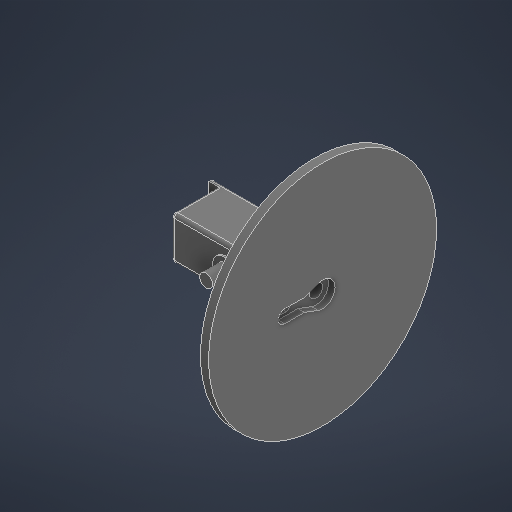
# Autodesk Inventor part: arm_MALE_full_size
Saved by Autodesk Inventor 2026.1 (Build 301233000, 233)
## iProperties
Created: 2025-10-10
Part Number: arm_MALE_full_size
Material: Generic
Document SubType Name: Modeling
Designer: Ethan
Density: 1 g/cm^3
Appearance: Gray
Author: Ethan
Autodesk Inventor part; units mm, degrees
ref_plane "YZ Plane" through (0, 0, 0) normal (1, 0, 0) x (0, 1, 0)
ref_plane "XZ Plane" through (0, 0, 0) normal (0, 1, 0) x (-1, 0, 0)
ref_plane "XY Plane" through (0, 0, 0) normal (0, 0, 1) x (1, 0, 0)
sketch "Sketch1" plane through (0, 0, 0) normal (0, 0, 1) x (1, 0, 0)
  line L0 (0, 0) -> (-40.25, 0)
  line L1 (-40.25, 0) -> (-40.25, 20.25)
  line L2 (-40.25, 20.25) -> (0, 20.25)
  line L3 (0, 20.25) -> (0, 0)
  dimension "d0" = 40.25
  dimension "d1" = 20.25
  constraints: 8 end point, 2 parallel, 1 horizontal, 1 perpendicular
  measures "d0" distance of L1.end L2.end
  measures "d1" distance of L0.end L1.end
extrude "Extrusion1" add sketch "Sketch1" along normal blind 3
sketch "Sketch2" plane through (0, 0, 3) normal (0, 0, 1) x (1, 0, 0)
  line L0 (0, 20.25) -> (-40.25, 20.25) projected
  line L1 (0, 20.25) -> (3, 20.25)
  line L2 (3, 20.25) -> (3, 14.125)
  line L3 (3, 14.125) -> (0, 14.125)
  line L4 (0, 14.125) -> (0, 20.25)
  line L5 (0, 0) -> (3, 0)
  line L6 (3, 0) -> (3, 6.125)
  line L7 (3, 6.125) -> (0, 6.125)
  line L8 (0, 6.125) -> (0, 0)
  line L9 (3, 20.25) -> (-40.25, 20.25)
  line L10 (-40.25, 20.25) -> (-40.25, 23.25)
  line L11 (-40.25, 23.25) -> (3, 23.25)
  line L12 (3, 23.25) -> (3, 20.25)
  line L13 (-40.25, 20.25) -> (-40.25, 0) projected
  line L14 (-40.25, 0) -> (-43.25, 0)
  line L15 (-43.25, 0) -> (-43.25, 23.25)
  line L16 (-43.25, 23.25) -> (-40.25, 23.25)
  line L17 (-40.25, 23.25) -> (-40.25, 0)
  line L18 (-43.25, 0) -> (3, 0)
  line L19 (3, 0) -> (3, -3)
  line L20 (3, -3) -> (-43.25, -3)
  line L21 (-43.25, -3) -> (-43.25, 0)
  point P0 (1.5, 6.125)
  dimension "d4" = 8
  dimension "d5" = 6.125
  dimension "d6" = 6.125
  dimension "d7" = 3
  dimension "d8" = 3
  dimension "d9" = 3
  dimension "d10" = 3
  dimension "d11" = 3
  constraints: 40 end point, 10 parallel, 5 horizontal, 5 perpendicular, 1 midpoint
  measures "d4" distance from line of L3 point (1.5, 6.125)
  measures "d5" distance of L1.end L2.end
  measures "d6" distance of L5.end L6.end
  measures "d7" distance between parallel lines of L4 L2
  measures "d8" distance between parallel lines of L8 L6
  measures "d9" distance between parallel lines of L0 L11
  measures "d10" distance between parallel lines of L13 L15
  measures "d11" distance between parallel lines of L18 L20
extrude "Extrusion2" add sketch "Sketch2" against normal blind 18
sketch "Sketch3" plane through (0, 0, -15) normal (0, 0, -1) x (-1, 0, 0)
  line L0 (-3, 23.25) -> (-3, 14.125) projected
  line L1 (43.25, -3) -> (43.25, 23.25) projected
  line L2 (-3, 23.25) -> (43.25, 23.25)
  line L3 (43.25, 23.25) -> (43.25, 20.25)
  line L4 (43.25, 20.25) -> (-3, 20.25)
  line L5 (-3, 20.25) -> (-3, 23.25)
  line L6 (0, 20.25) -> (40.25, 20.25) projected
  line L7 (-3, -3) -> (-3, 6.125) projected
  line L8 (-3, 0) -> (43.25, 0)
  line L9 (43.25, 0) -> (43.25, -3)
  line L10 (43.25, -3) -> (-3, -3)
  line L11 (-3, -3) -> (-3, 0)
  point P0 (0, 0)
  point P1 (-3, 20.25)
  dimension "d14" = 0
  constraints: 16 end point, 4 parallel, 2 horizontal, 2 perpendicular, 2 point on line
  measures "d14" distance between parallel lines of L6 L4
extrude "Extrusion3" add sketch "Sketch3" along normal blind 13
sketch "Sketch4" plane through (-43.25, -3, 3) normal (-1, 0, 0) x (0, 0, 1)
  line L0 (0, 0) -> (-31, 0) projected
  line L1 (-31, 26.25) -> (-28, 26.25)
  line L2 (-28, 26.25) -> (-28, 0)
  line L3 (-28, 0) -> (-31, 0)
  line L4 (-31, 0) -> (-31, 26.25)
  line L5 (0, 26.25) -> (-31, 26.25) projected
  point P0 (-3, 3)
  dimension "d17" = 3
  dimension "d18" = 0
  constraints: 8 end point, 2 parallel, 1 horizontal, 1 perpendicular, 1 point on line
  measures "d17" distance from line of L1.start L2
  measures "d18" distance between parallel lines of L1 L5
extrude "Extrusion4" add sketch "Sketch4" against normal blind 3
sketch "Sketch5" plane through (-43.25, -3, 3) normal (-1, 0, 0) x (0, 0, 1)
  line L0 (0, 26.25) -> (-31, 26.25) projected
  line L1 (0, 0) -> (-31, 0) projected
  line L2 (-31, 26.25) -> (-28, 26.25)
  line L3 (-28, 26.25) -> (-28, 0)
  line L4 (-28, 0) -> (-31, 0)
  line L5 (-31, 0) -> (-31, 26.25)
  line L6 (-28, 3) -> (-28, 23.25) projected
  point P0 (-3, 3)
  dimension "d21" = 0
  constraints: 8 end point, 2 parallel, 1 horizontal, 1 perpendicular, 1 point on line
  measures "d21" distance between parallel lines of L6 L3
extrude "Extrusion5" add sketch "Sketch5" along normal blind 5
sketch "Sketch6" plane through (0, 0, -28) normal (0, 0, -1) x (-1, 0, 0)
  circle A0 centre (44.55, 17.25) radius 2.5
  circle A1 centre (44.55, 3) radius 2.5
  line L0 (-3, 23.25) -> (48.25, 23.25) projected
  line L1 (-3, -3) -> (48.25, -3) projected
  line L2 (40.25, 0) -> (40.25, 20.25) projected
  line L3 (42.05, 17.25) -> (47.05, 17.25)
  line L4 (47.05, 17.25) -> (47.05, 3)
  line L5 (47.05, 3) -> (42.05, 3)
  line L6 (42.05, 3) -> (42.05, 17.25)
  point P0 (0, 0)
  point P1 (42.05, 3)
  point P2 (42.05, 3)
  point P3 (46.4709, 4.6)
  dimension "d26" = 5
  dimension "d27" = 5
  dimension "d24" = 6
  dimension "d25" = 6
  dimension "d28" = 4.3
  dimension "d29" = 4.3
  constraints: 8 end point, 2 parallel, 2 vertical, 1 horizontal, 1 perpendicular, 6 other
  measures "d24" distance from line of L0 point (44.55, 17.25)
  measures "d25" distance from line of L1 point (44.55, 3)
  measures "d28" distance from line of L2 point (44.55, 17.25)
  measures "d29" distance from line of L2 point (44.55, 3)
extrude "Extrusion6" cut sketch "Sketch6" against normal blind 3
sketch "Sketch7" plane through (-43.25, -3, 3) normal (-1, 0, 0) x (0, 0, 1)
  line L0 (-18, 23.25) -> (-31, 23.25) projected
  line L1 (-3, 3) -> (-18, 3) projected
  line L2 (-18, 23.25) -> (-11, 23.25)
  line L3 (-11, 23.25) -> (-11, 3)
  line L4 (-11, 3) -> (-18, 3)
  line L5 (-18, 3) -> (-18, 23.25)
  line L6 (-28, 0) -> (-28, 26.25) projected
  dimension "d38" = 17
  constraints: 8 end point, 2 parallel, 1 horizontal, 1 perpendicular, 1 point on line
  measures "d38" distance between parallel lines of L6 L3
extrude "Extrusion7" cut sketch "Sketch7" against normal blind 3
sketch "Sketch8" plane through (0, 0, 3) normal (0, 0, 1) x (1, 0, 0)
  line L0 (0, 6.125) -> (0, 14.125) projected
  line L1 (-43.25, -3) -> (3, -3) projected
  line L2 (3, 23.25) -> (-43.25, 23.25) projected
  circle A0 centre (-10, 10) radius 7
  point P0 (0, 0)
  point P1 (0, 10.125)
  point P2 (-2, 5)
  point P3 (-15, 2)
  point P4 (-18, 15)
  dimension "d69" = 14
  constraints: 1 centre point, 1 midpoint
  measures "d69" diameter of A0
extrude "Extrusion8" add sketch "Sketch8" along normal blind 1
sketch "Sketch11" plane through (-10, 10, 4) normal (0, 0, 1) x (1, 0, 0)
  circle A0 centre (0, 0) radius 3.97
  point P0 (10, -10)
  dimension "d70" = 7.94
  constraints: 1 centre point
  measures "d70" diameter of A0
extrude "Extrusion10" add sketch "Sketch11" along normal blind 11
fillet "Fillet1" radius 2 7 edges at (-20.125, -3, 3) (-20.125, 23.25, 3) (-43.25, 10.125, 3) (-22.625, 23.25, -28) (-22.625, -3, -28) (-43.25, -3, -11) (-43.25, 23.25, -11)
sketch "Sketch12" plane through (3, 14.125, -13) normal (1, 0, 0) x (0, 0, -1)
  arc A0 (15, 7.125) -> (13, 9.125) centre (13, 7.125) ccw projected
  line L0 (15, 7.125) -> (-16, 7.125)
  line L1 (-16, 7.125) -> (-16, 9.125)
  line L2 (-16, 9.125) -> (15, 9.125)
  line L3 (15, 9.125) -> (15, 7.125)
  line L4 (-16, 7.125) -> (-16, 0) projected
  line L5 (-14, -15.125) -> (-16, -15.125) projected
  line L6 (-16, -15.125) -> (15, -15.125)
  line L7 (15, -15.125) -> (15, -17.125)
  line L8 (15, -17.125) -> (-16, -17.125)
  line L9 (-16, -17.125) -> (-16, -15.125)
  line L10 (-14, -17.125) -> (13, -17.125) projected
  line L11 (15, 7.125) -> (15, -15.125) projected
  line L12 (-16, 7.125) -> (15, 7.125)
  line L13 (15, 7.125) -> (15, 0)
  line L14 (15, 0) -> (-16, 0)
  line L15 (-16, 0) -> (-16, 7.125)
  line L16 (15, -11.125) -> (15, 3.125) projected
  line L17 (-16, -15.125) -> (15, -15.125)
  line L18 (15, -15.125) -> (15, -8)
  line L19 (15, -8) -> (-16, -8)
  line L20 (-16, -8) -> (-16, -15.125)
  line L21 (-16, -8) -> (2, -8) projected
  point P0 (-13, -14.125)
  point P1 (-16, 8.125)
  point P2 (15, -8)
  dimension "d74" = 0
  dimension "d75" = 0
  dimension "d107" = 2
  dimension "d108" = 0
  constraints: 32 end point, 8 parallel, 4 horizontal, 4 perpendicular, 2 point on line, 1 midpoint
  measures "d74" distance from line of L4 point (-16, 8.125)
  measures "d75" distance between parallel lines of L10 L8
  measures "d107" distance between parallel lines of L2 L0
  measures "d108" distance between parallel lines of L19 L21
ref_plane "Work Plane1" through (23, 14.125, -15) normal (1, 0, 0) x (0, 0, -1)
extrude "Extrusion14" add sketch "Sketch12" along normal blind 20
fillet "Fillet2" radius 2 4 edges at (13, 23.25, 3) (13, 23.25, -28) (13, -3, 3) (13, -3, -28)
sketch "Sketch19" plane through (23, 14.125, -13) normal (1, 0, 0) x (0, 0, -1)
  line L0 (-16, 11.5) -> (15, 11.5)
  line L1 (15, 11.5) -> (15, -19.5)
  line L2 (15, -19.5) -> (-16, -19.5)
  line L3 (-16, -19.5) -> (-16, 11.5)
  line L4 (15, 0) -> (15, 7.125) projected
  line L5 (-14, -17.125) -> (13, -17.125) projected
  line L6 (-13, -8) -> (-13, 0) projected
  circle A0 centre (0.0561, -4) radius 69.5
  point P0 (-13, -14.125)
  point P1 (-13, -4)
  dimension "d110" = 0
  dimension "d126" = 15.5
  dimension "d127" = 15.5
  dimension "d136" = 139
  constraints: 8 end point, 2 parallel, 1 centre point, 1 horizontal, 1 midpoint, 1 perpendicular
  measures "d110" distance between parallel lines of L1 L4
  measures "d126" distance from line of point (-13, -4) L0
  measures "d127" distance from line of point (-13, -4) L2
  measures "d136" diameter of A0
extrude "Extrusion15" add sketch "Sketch19" along normal blind 10 contours L0 L1 L2 L3 | A0
sketch "Sketch23" plane through (33, 10.125, -13.0561) normal (1, 0, 0) x (0, 0, -1)
  circle A0 centre (0, 0) radius 7.6
  circle A1 centre (-23.1337, 0) radius 3.925
  line L0 (-23.1337, -3.925) -> (-6.508, -3.925)
  line L1 (-23.1337, 3.925) -> (-6.508, 3.925)
  line L2 (-11.0587, -3.925) -> (-2.7018, -7.1035)
  line L3 (-11.0587, 3.925) -> (-2.7018, 7.1035)
  circle A2 centre (0, 0) radius 69.5 projected
  line L4 (7.6, 0) -> (-27.0587, 0)
  point P0 (-13.0561, -10.125)
  dimension "d137" = 15.2
  dimension "d138" = 7.85
  dimension "d139" = 0
  dimension "d140" = 16
  dimension "d141" = 16
  constraints: 10 end point, 8 point on circle, 2 centre point, 2 horizontal, 2 point on line, 2 tangent, 1 concentric, 1 parallel
  measures "d137" diameter of A0
  measures "d138" diameter of A1
  measures "d139" vertical distance of A0.centre A1.centre
  measures "d140" horizontal distance of L4.end L2.start
  measures "d141" horizontal distance of L4.end L3.start
extrude "Extrusion19" cut sketch "Sketch23" against normal blind 4 contours L4 A0 | A0 L4 | A0 L1 L3 | L2 L0 A0 | L4 A1 L1 A0 | A0 L0 A1 L4 | L4 A1 | A1 L4
sketch "Sketch24" plane through (29, 10.125, -13.0561) normal (1, 0, 0) x (0, 0, -1)
  circle A0 centre (-23.1337, 0) radius 2
  line L0 (-17.0561, 6.875) -> (-17.0561, -7.125) projected
  arc A1 (-23.1337, 3.925) -> (-23.1337, -3.925) centre (-23.1337, 0) ccw projected
  circle A2 centre (-18.1337, 0) radius 2
  line L1 (-23.1337, -2) -> (-18.1337, -2)
  line L2 (-18.1337, 2) -> (-23.1337, 2)
  point P0 (-13.0561, -10.125)
  dimension "d144" = 4
  dimension "d146" = 4
  dimension "d147" = 5
  constraints: 4 end point, 4 point on circle, 2 centre point, 1 concentric, 1 horizontal, 1 tangent
  measures "d144" diameter of A0
  measures "d146" diameter of A2
  measures "d147" distance of A2.centre A0.centre
extrude "Extrusion20" cut sketch "Sketch24" against normal blind 10
sketch "Sketch25" plane through (29, 10.125, -13.0561) normal (1, 0, 0) x (0, 0, -1)
  circle A0 centre (0, 0) radius 4
  point P0 (-13.0561, -10.125)
  dimension "d150" = 8
  constraints: 1 centre point
  measures "d150" diameter of A0
extrude "Extrusion21" cut sketch "Sketch25" against normal blind 10
sketch "Sketch26" plane through (23, 10.125, -13.0561) normal (-1, 0, 0) x (0, 0, 1)
  circle A0 centre (0, 0) radius 4 projected
  circle A1 centre (0, 0) radius 34.5
  circle A2 centre (0, 0) radius 69.5 projected
  arc A3 (2.7018, 7.1035) -> (2.7018, -7.1035) centre (0, 0) ccw projected
  circle A4 centre (0, 0) radius 69.5
  point P0 (13.0561, -10.125)
  dimension "d153" = 35
  constraints: 2 centre point, 2 coincident, 1 concentric
  measures "d153" radial gap between concentric circles of A2 A1
extrude "Extrusion22" cut sketch "Sketch26" against normal blind 5 contours A2
body "Solid1"
